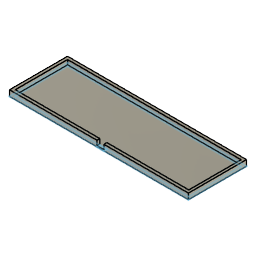
Klawiatura (Autodesk Fusion 360 design; units mm, degrees)
part number: 2025-11-11-11-56-58-559
Autodesk Fusion 360 part; units mm, degrees
sketch "Szkic1" plane through (0, 0, 0) normal (0, 0, 1) x (1, 0, 0)
  line L0 (-39.0522, 48.0519) -> (259.5478, 48.0519)
  line L1 (259.5478, 48.0519) -> (259.5478, -41.9481)
  line L2 (259.5478, -41.9481) -> (-39.0522, -41.9481)
  line L3 (-39.0522, -41.9481) -> (-39.0522, 48.0519)
  line L4 (-44.0522, 53.0519) -> (263.9478, 53.0519)
  line L5 (263.9478, 53.0519) -> (263.9478, -46.9481)
  line L6 (263.9478, -46.9481) -> (-44.0522, -46.9481)
  line L7 (-44.0522, -46.9481) -> (-44.0522, 53.0519)
  line L8 (118.5478, -41.9481) -> (106.5478, -41.9481)
  line L9 (106.5478, -41.9481) -> (106.5478, -46.9481)
  line L10 (106.5478, -46.9481) -> (118.5478, -46.9481)
  line L11 (118.5478, -46.9481) -> (118.5478, -41.9481)
  dimension "d1" = 298.6
  dimension "d2" = 90
  dimension "d3" = 308
  dimension "d4" = 100
  dimension "d5" = 5
  dimension "d6" = 5
  dimension "d7" = 141
  dimension "d8" = 12
  constraint horizontal L0
  constraint vertical L1
  constraint horizontal L2
  constraint vertical L3
  constraint horizontal L4
  constraint vertical L5
  constraint horizontal L6
  constraint vertical L7
  constraint horizontal L8
  constraint vertical L9
  constraint horizontal L10
  constraint vertical L11
  constraint coincident L6 L9.end
  constraint coincident L2 L8.start
  measures "d1" distance of L0.start L0.end
  measures "d2" distance of L0.start L2.end
  measures "d3" distance of L4.start L4.end
  measures "d4" distance of L4.start L6.end
  measures "d5" distance of L0 L4
  measures "d6" distance of L3 L7
  measures "d7" distance of L1.end L11
  measures "d8" distance of L8.start L8.end
extrude "Wyciągnięcie proste1" add sketch "Szkic1" along normal blind 5 contours L0 L1 L2 L3 L4 L5 L6 L7 L9 L11
extrude "Wyciągnięcie proste2" add sketch "Szkic1" along normal blind 2 contours L0 L1 L2 L3 L8
extrude "Wyciągnięcie proste3" add sketch "Szkic1" along normal blind 2 contours L2 L6 L8 L9 L10 L11
extrude "Wyciągnięcie proste4" add 1 faces at (60.2811, 51.3852, 5) along direction (0, 0, 1) blind 5
